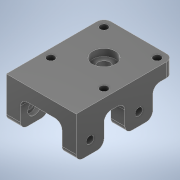
# Autodesk Inventor part: Shoulderbottom
Saved by Autodesk Inventor 2022 (Build 260153000, 153)
## iProperties
Created: 2022-03-24
Part Number: Shoulderbottom
Material: Genérico
Document SubType Name: Modeling
Designer: JK
Density: 1 g/cm^3
Appearance: Suave - Negro
Author: JK
Autodesk Inventor part; units mm, degrees
ref_plane "YZ Plane" through (0, 0, 0) normal (1, 0, 0) x (0, 1, 0)
ref_plane "XZ Plane" through (0, 0, 0) normal (0, 1, 0) x (-1, 0, 0)
ref_plane "XY Plane" through (0, 0, 0) normal (0, 0, 1) x (1, 0, 0)
sketch "Boceto1" plane through (0, 0, 0) normal (0, 1, 0) x (-1, 0, 0)
  line L0 (-24.9, 24.85) -> (24.9, 24.85)
  line L1 (24.9, 24.85) -> (24.9, -24.85)
  line L2 (24.9, -24.85) -> (-24.9, -24.85)
  line L3 (-24.9, -24.85) -> (-24.9, 24.85)
  line L4 (-24.9, 24.85) -> (24.9, -24.85) construction
  line L5 (24.9, 24.85) -> (-24.9, -24.85) construction
  circle A0 centre (0, 0) radius 4.35
  dimension "d0" = 49.8
  dimension "d1" = 8.7
  dimension "d2" = 49.7
  constraints: 12 end point, 2 midpoint, 2 parallel, 1 centre point, 1 coincident, 1 horizontal, 1 perpendicular
  measures "d0" distance of L0.start L0.end
  measures "d1" diameter of A0
  measures "d2" distance of L0.end L1.end
extrude "Extrusión1" add sketch "Boceto1" along normal blind 10
sketch "Boceto4" plane through (0, 0, 0) normal (0, -1, 0) x (1, 0, 0)
  line L0 (24.9, 24.85) -> (24.9, -24.85) projected
  line L1 (-24.9, -24.85) -> (-24.9, 24.85) projected
  line L2 (24.9, 24.85) -> (-24.9, 24.85)
  line L3 (-24.9, 24.85) -> (-24.9, 17.85)
  line L4 (-24.9, 17.85) -> (24.9, 17.85)
  line L5 (24.9, 17.85) -> (24.9, 24.85)
  line L6 (24.9, -24.85) -> (-24.9, -24.85) projected
  line L7 (24.9, -24.85) -> (-24.9, -24.85)
  line L8 (-24.9, -24.85) -> (-24.9, -17.85)
  line L9 (-24.9, -17.85) -> (24.9, -17.85)
  line L10 (24.9, -17.85) -> (24.9, -24.85)
  line L11 (24.9, -24.85) -> (-24.9, -24.85) projected
  line L12 (24.9, 24.85) -> (24.9, -24.85) projected
  line L13 (-24.9, 24.85) -> (24.9, 24.85) projected
  line L14 (-24.9, -24.85) -> (-24.9, 24.85) projected
  circle A0 centre (0, 0) radius 4.35 projected
  point P0 (-24.9, -17.85)
  point P1 (24.9, -17.85)
  dimension "d14" = 7
  dimension "d15" = 7
  constraints: 16 end point, 4 parallel, 2 horizontal, 2 perpendicular, 2 point on line
  measures "d14" distance between parallel lines of L4 L2
  measures "d15" distance between parallel lines of L6 L9
extrude "Extrusión4" [suppressed]
sketch "Boceto5" plane through (0, 0, 0) normal (0, 0, 1) x (1, 0, 0)
  circle A0 centre (17.9, -5.5) radius 2.7
  circle A1 centre (-17.9, -5.5) radius 2.7
  line L0 (20, -12) -> (-20, -12) projected
  line L1 (24.9, 0) -> (24.9, 10) projected
  line L2 (-24.9, 0) -> (-24.9, 10) projected
  point P0 (0, 0)
  point P1 (-24.9, 10)
  dimension "d19" = 6.5
  dimension "d20" = 5.4
  dimension "d21" = 7
  dimension "d22" = 7
  constraints: 2 centre point, 1 equal radius, 1 horizontal alignment, 2 other
  measures "d19" distance from line of L0 A0.centre
  measures "d20" diameter of A0
extrude "Extrusión5" [suppressed]
sketch "Boceto6" plane through (0, 0, 0) normal (0, 0, 1) x (1, 0, 0)
  circle A0 centre (13, -5.5) radius 2.7 projected
  circle A1 centre (13, -5.5) radius 4.65
  circle A2 centre (-13, -5.5) radius 2.7 projected
  circle A3 centre (-13, -5.5) radius 4.65
  point P0 (0, 0)
  dimension "d25" = 9.3
  constraints: 2 centre point, 2 coincident, 1 equal radius
  measures "d25" diameter of A1
extrude "Extrusión6" [suppressed]
fillet "Empalme2" [suppressed]
fillet "Empalme3" [suppressed]
sketch "Boceto8" plane through (0, 0, 0) normal (0, -1, 0) x (1, 0, 0)
  circle A0 centre (0, 0) radius 4.35 projected
  line L0 (-24.9, -24.85) -> (-24.9, 24.85) projected
  line L1 (24.9, 24.85) -> (24.9, -24.85) projected
  circle A1 centre (0, 0) radius 7.5
  line L2 (24.9, -24.85) -> (-24.9, -24.85) projected
  line L3 (-24.9, 24.85) -> (24.9, 24.85) projected
  dimension "d30" = 15
  constraints: 1 centre point, 1 coincident
  measures "d30" diameter of A1
extrude "Extrusión7" [suppressed]
fillet "Empalme4" [suppressed]
sketch "Boceto9" plane through (0, 10, 0) normal (0, 1, 0) x (1, 0, 0)
  circle A0 centre (0, 0) radius 8.125
  dimension "d34" = 16.25
  constraints: 1 centre point, 1 coincident
  measures "d34" diameter of A0
extrude "Extrusión8" cut sketch "Boceto9" against normal blind 5
sketch "Boceto10" plane through (0, 0, 0) normal (0, -1, 0) x (1, 0, 0)
  circle A0 centre (19, -19) radius 2.7 projected
  circle A1 centre (-19, -19) radius 2.7 projected
  circle A2 centre (19, 19) radius 2.7 projected
  circle A3 centre (-19, 19) radius 2.7 projected
  point P0 (0, 0)
extrude "Extrusión9" cut sketch "Boceto10" against normal through all
fillet "Empalme5" radius 5 4 edges at (-24.9, 5, 24.85) (24.9, 5, 24.85) (24.9, 5, -24.85) (-24.9, 5, -24.85)
sketch "Boceto11" plane through (0, 0, 0) normal (0, -1, 0) x (1, 0, 0)
  circle A0 centre (19, 19) radius 2.7 projected
  circle A1 centre (19, 19) radius 4.05
  line L0 (14.95, 16.6617) -> (14.95, 21.3383)
  line L1 (14.95, 21.3383) -> (19, 23.6765)
  line L2 (19, 23.6765) -> (23.05, 21.3383)
  line L3 (23.05, 21.3383) -> (23.05, 16.6617)
  line L4 (23.05, 16.6617) -> (19, 14.3235)
  line L5 (19, 14.3235) -> (14.95, 16.6617)
  point P0 (0, 0)
  dimension "d40" = 8.1
  constraints: 12 end point, 2 coincident, 1 centre point, 1 tangent, 1 vertical, 13 other
  measures "d40" diameter of A1
extrude "Extrusión10" cut sketch "Boceto11" against normal blind 4 contours A0 | A1 | L3 L4 A1 | A1 L2 L3 | A1 L1 L2 | L4 L5 A1 | A1 L0 L1 | L5 L0 A1
pattern_circular "Patrón circular1" count 4 over 360 about axis through (0, 0, 0) along (0, 1, 0) of "Extrusión10"
sketch "Boceto12" plane through (0, 0, 0) normal (0, -1, 0) x (1, 0, 0)
  line L0 (-24.9, -19.85) -> (-24.9, 19.85) projected
  line L1 (-24.9, 10) -> (-14.9, 10)
  line L2 (-14.9, 10) -> (-14.9, -10)
  line L3 (-14.9, -10) -> (-24.9, -10)
  line L4 (-24.9, -10) -> (-24.9, 10)
  line L5 (24.9, 19.85) -> (24.9, -19.85) projected
  line L6 (24.9, 10) -> (14.9, 10)
  line L7 (14.9, 10) -> (14.9, -10)
  line L8 (14.9, -10) -> (24.9, -10)
  line L9 (24.9, -10) -> (24.9, 10)
  point P0 (0, 0)
  point P1 (24.9, -10)
  point P2 (-24.9, -10)
  dimension "d46" = 20
  dimension "d47" = 10
  dimension "d48" = 10
  dimension "d49" = 10
  constraints: 16 end point, 4 parallel, 2 collinear, 2 horizontal, 2 perpendicular, 2 point on line
  measures "d46" distance between parallel lines of L1 L3
  measures "d47" distance from line of point (0, 0) L1
  measures "d48" distance of L1.start L1.end
  measures "d49" distance of L6.start L6.end
extrude "Extrusión11" add sketch "Boceto12" along normal blind 20
sketch "Boceto13" plane through (-24.9, 0, -19.85) normal (-1, 0, 0) x (0, 0, 1)
  circle A0 centre (19.85, -11) radius 2.7
  point P0 (19.85, 0)
  dimension "d52" = 5.4
  dimension "d53" = 11
  constraints: 1 centre point
  measures "d52" diameter of A0
  measures "d53" distance of A0.centre point (19.85, 0)
extrude "Extrusión12" cut sketch "Boceto13" against normal through all
fillet "Empalme6" radius 5 6 edges at (-19.9, 0, -10) (-14.9, 0, 0) (19.9, 0, -10) (14.9, 0, 0) (19.9, 0, 10) (-19.9, 0, 10)
fillet "Empalme7" radius 5 4 edges at (-19.9, -20, -10) (-19.9, -20, 10) (19.9, -20, -10) (19.9, -20, 10)
sketch "Boceto15" plane through (0, 0, 0) normal (1, 0, 0) x (0, 1, 0)
  circle A0 centre (-11, 0) radius 2.7 projected
  circle A1 centre (-11, 0) radius 4.7
  point P0 (0, 0)
  dimension "d58" = 9.4
  constraints: 1 centre point, 1 coincident
  measures "d58" diameter of A1
extrude "Extrusión13" cut sketch "Boceto15" along normal mid plane 36 contours A0 | A1
sketch "Boceto16" plane through (0, 0, 0) normal (0, -1, 0) x (1, 0, 0)
  line L0 (-9.9, -15) -> (-9.9, 15) projected
  arc A0 (-24.9, -19.85) -> (-19.9, -24.85) centre (-19.9, -19.85) ccw projected
  line L1 (-24.9, -19.85) -> (-24.9, 19.85) projected
  arc A1 (-19.9, 24.85) -> (-24.9, 19.85) centre (-19.9, 19.85) ccw projected
  line L2 (-19.9, 24.85) -> (19.9, 24.85) projected
  arc A2 (24.9, 19.85) -> (19.9, 24.85) centre (19.9, 19.85) ccw projected
  line L3 (24.9, 19.85) -> (24.9, -19.85) projected
  arc A3 (19.9, -24.85) -> (24.9, -19.85) centre (19.9, -19.85) ccw projected
  line L4 (19.9, -24.85) -> (-19.9, -24.85) projected
  circle A4 centre (-19, 19) radius 2.7 projected
  circle A5 centre (-19, -19) radius 2.7 projected
  circle A6 centre (19, 19) radius 2.7 projected
  circle A7 centre (19, -19) radius 2.7 projected
  circle A8 centre (0, 0) radius 8.125 projected
  line L5 (-24.9, -19.85) -> (-24.9, 19.85) projected
  line L6 (-24.9, 24.85) -> (24.9, 24.85)
  line L7 (24.9, 24.85) -> (24.9, 44.85)
  line L8 (24.9, 44.85) -> (-24.9, 44.85)
  line L9 (-24.9, 44.85) -> (-24.9, 24.85)
  line L10 (24.9, 19.85) -> (24.9, -19.85) projected
  line L11 (-19.9, 24.85) -> (19.9, 24.85) projected
  arc A9 (-19.9, 24.85) -> (-24.9, 19.85) centre (-19.9, 19.85) ccw projected
  line L12 (-24.9, 19.85) -> (24.9, 19.85)
  line L13 (24.9, 19.85) -> (24.9, 24.85)
  line L14 (24.9, 24.85) -> (-24.9, 24.85)
  line L15 (-24.9, 24.85) -> (-24.9, 19.85)
  point P0 (-24.9, 19.85)
  dimension "d64" = 20
  constraints: 16 end point, 4 parallel, 2 collinear, 2 horizontal, 2 perpendicular, 1 point on circle, 1 point on line
  measures "d64" distance of L8.end L6.start
extrude "Extrusión14" add sketch "Boceto16" against normal up to surface (10 mm away) contours L15 L6 A1 | L6 L9 L8 L7 L2 | L6 L13 A2
sketch "Boceto18" plane through (0, 0, 0) normal (0, -1, 0) x (1, 0, 0)
  line L0 (-24.9, 44.85) -> (-24.9, 15) projected
  line L1 (-24.9, 44.85) -> (-14.9, 44.85)
  line L2 (-14.9, 44.85) -> (-14.9, 24.85)
  line L3 (-14.9, 24.85) -> (-24.9, 24.85)
  line L4 (-24.9, 24.85) -> (-24.9, 44.85)
  line L5 (24.9, 44.85) -> (24.9, -19.85) projected
  line L6 (24.9, 44.85) -> (14.9, 44.85)
  line L7 (14.9, 44.85) -> (14.9, 24.85)
  line L8 (14.9, 24.85) -> (24.9, 24.85)
  line L9 (24.9, 24.85) -> (24.9, 44.85)
  line L10 (-14.9, -5) -> (-14.9, 5) projected
  line L11 (14.9, 5) -> (14.9, -5) projected
  point P0 (0, 0)
  point P1 (24.9, 24.85)
  dimension "d69" = 20
  constraints: 16 end point, 4 parallel, 3 collinear, 2 horizontal, 2 perpendicular
  measures "d69" distance between parallel lines of L1 L3
extrude "Extrusión15" add sketch "Boceto18" along normal up to surface (20 mm away)
fillet "Empalme8" radius 5 4 edges at (19.9, 0, 24.85) (14.9, 0, 34.85) (-14.9, 0, 34.85) (-19.9, 0, 24.85)
fillet "Empalme9" radius 5 4 edges at (-19.9, -20, 24.85) (19.9, -20, 24.85) (-19.9, -20, 44.85) (19.9, -20, 44.85)
sketch "Boceto19" plane through (24.9, 0, -19.85) normal (1, 0, 0) x (0, 0, -1)
  circle A0 centre (-54.7, -11) radius 2.7
  line L0 (-64.7, 10) -> (-64.7, -15) projected
  circle A1 centre (-19.85, -11) radius 2.7 projected
  point P0 (-19.85, 0)
  dimension "d74" = 5.4
  dimension "d75" = 10
  constraints: 1 centre point, 1 horizontal alignment
  measures "d74" diameter of A0
  measures "d75" distance from line of L0 A0.centre
extrude "Extrusión16" cut sketch "Boceto19" against normal through all contours A0
sketch "Boceto20" plane through (0, 0, 0) normal (1, 0, 0) x (0, 1, 0)
  circle A0 centre (-11, 34.85) radius 2.7 projected
  circle A1 centre (-11, 34.85) radius 4.7
  point P0 (0, 0)
  dimension "d78" = 9.4
  constraints: 1 centre point, 1 coincident
  measures "d78" diameter of A1
extrude "Extrusión17" cut sketch "Boceto20" along normal mid plane 36 contours A0 | A1
